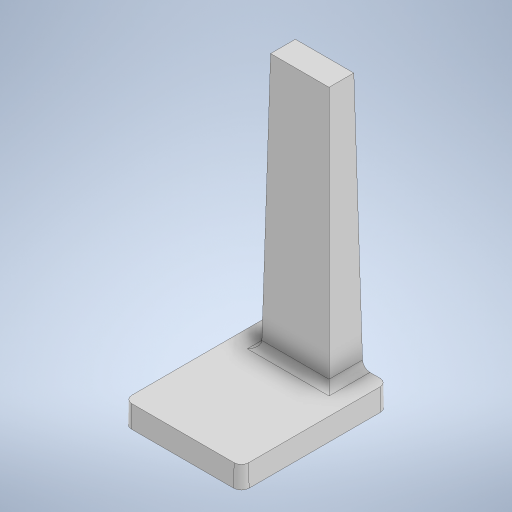
# Autodesk Inventor part: Based Cast Image
Saved by Autodesk Inventor 2023 (Build 270158000, 158)
## iProperties
Created: 2022-12-28
Part Number: Based Cast Image
Material: Generic
Document SubType Name: Modeling
Designer: tgr41
Density: 1 g/cm^3
Appearance: Default
Author: tgr41
Autodesk Inventor part; units mm, degrees
ref_plane "YZ Plane" through (0, 0, 0) normal (1, 0, 0) x (0, 1, 0)
ref_plane "XZ Plane" through (0, 0, 0) normal (0, 1, 0) x (-1, 0, 0)
ref_plane "XY Plane" through (0, 0, 0) normal (0, 0, 1) x (1, 0, 0)
sketch "Sketch1" plane through (0, 0, 0) normal (1, 0, 0) x (0, 1, 0)
  line L0 (0, 0) -> (111.125, 0)
  line L1 (111.125, 0) -> (111.125, -12.7)
  line L2 (111.125, -12.7) -> (-9.525, -12.7)
  line L3 (-9.525, -12.7) -> (-9.525, 50.8)
  line L4 (-9.525, 50.8) -> (0, 50.8)
  line L5 (0, 50.8) -> (0, 0)
  line L6 (0, 0) -> (0, -12.7)
  dimension "d0" = 111.125
  dimension "d1" = 12.7
  dimension "d2" = 120.65
  dimension "d3" = 63.5
  constraints: 14 end point, 5 perpendicular, 1 horizontal, 1 point on line, 1 vertical
  measures "d0" distance of L0.start L0.end
  measures "d1" distance of L0.end L1.end
  measures "d2" distance of L1.end L2.end
  measures "d3" distance of L2.end L3.end
extrude "Extrusion1" add sketch "Sketch1" along normal blind 25.4 contours L0 L1 L2 L6
extrude "Extrusion3" add sketch "Sketch1" along normal blind 38.1 and the other way blind 12.7 contours L6 L2 L3 L4 L5
fillet "Fillet2" radius 3.175 4 edges at (38.1, -4.7625, -12.7) (38.1, -4.7625, 50.8) (-12.7, -4.7625, 50.8) (-12.7, -4.7625, -12.7)
draft "FaceDraft1" angle 1 pull direction (0, 1, 0) faces at (25.4, 37.0417, -4.2333) (8.4667, 74.0833, 0) (0, 37.0417, -4.2333) fixed edges at (25.4, 111.125, -6.35) (12.7, 111.125, 0) (0, 111.125, -6.35)
draft "FaceDraft2" angle 1 pull direction (0, 1, 0) faces at (38.1, -3.175, 28.575) (37.0845, -6.35, 49.9524) (36.085, -6.35, -12.4805) (5.2917, -3.175, 50.8) (8.4667, 37.0417, -12.7) (-12.5589, -3.175, 48.5608) (-12.6645, -6.35, -9.9982) (-12.7, -3.175, 28.575) fixed edges at (38.1, 0, 19.05) (37.1701, 0, 49.8701) (37.1701, 0, -11.7701) (12.7, 0, 50.8) (-5.7323, 0, -12.7) (31.1323, 0, -12.7) (-11.7701, 0, 49.8701) (-11.7701, 0, -11.7701) (-12.7, 0, 19.05)
fillet "Fillet3" radius 3.175 3 edges at (27.3397, 0, -5.3802) (12.7, 0, 1.9397) (-1.9397, 0, -5.3802)
body "Solid1"
